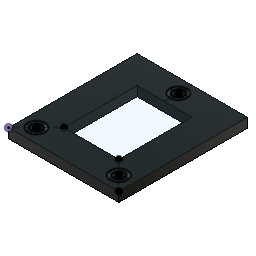
Combat Arrow Assembly v9 (Autodesk Fusion 360 archive; units mm, degrees)
design "Neoprene Clamp mk2"
Autodesk Fusion 360 part; units mm, degrees
sketch "Sketch1" plane through (0, 0, 0) normal (0, 0, 1) x (1, 0, 0)
  line L0 (0, 0) -> (38.354, 0)
  line L1 (38.354, 0) -> (38.354, 44.704)
  line L2 (38.354, 44.704) -> (0, 44.704)
  line L3 (0, 44.704) -> (0, 0)
  line L4 (28.702, 35.052) -> (9.652, 35.052)
  line L5 (9.652, 35.052) -> (9.652, 9.652)
  line L6 (9.652, 9.652) -> (28.702, 9.652)
  line L7 (28.702, 9.652) -> (28.702, 35.052)
  line L8 (28.702, 35.052) -> (9.652, 9.652) construction
  line L9 (9.652, 35.052) -> (28.702, 9.652) construction
  line L10 (19.177, 44.704) -> (19.177, 0) construction
  line L11 (0, 22.352) -> (38.354, 22.352) construction
  point P0 (19.177, 22.352)
  dimension "d13" = 38.354
  dimension "d14" = 44.704
  dimension "d15" = 19.05
  dimension "d16" = 25.4
  constraint horizontal L0
  constraint vertical L1
  constraint horizontal L2
  constraint vertical L3
  constraint coincident L0.start L3.end
  constraint horizontal L4
  constraint perpendicular L4 L5
  constraint parallel L4 L6
  constraint parallel L5 L7
  constraint coincident L8 P0
  constraint coincident L9 P0
  constraint midpoint L2 L10.start
  constraint midpoint L0 L10.end
  constraint midpoint L3 L11.start
  constraint midpoint L1 L11.end
  constraint coincident P0 L11
  constraint coincident P0 L10
  measures "d13" distance of L0.start L0.end
  measures "d14" distance of L0.start L2.end
  measures "d15" distance of L5.end L6.end
  measures "d16" distance of L4.start L6.end
extrude "Extrude1" add sketch "Sketch1" along normal blind 3.3528
sketch "Sketch2" plane through (0, 0, 3.3528) normal (0, 0, 1) x (-1, 0, 0)
  line L0 (-28.702, -35.052) -> (-28.702, -9.652)
  line L1 (-28.702, -9.652) -> (-9.652, -9.652)
  line L2 (-9.652, -9.652) -> (-9.652, -35.052)
  line L3 (-9.652, -35.052) -> (-28.702, -35.052)
  line L4 (0, -44.704) -> (0, 0)
  line L5 (0, 0) -> (-38.354, 0)
  line L6 (-38.354, 0) -> (-38.354, -44.704)
  line L7 (-38.354, -44.704) -> (0, -44.704)
  line L8 (-19.177, -35.052) -> (-19.177, -44.704) construction
  line L9 (-9.652, -9.652) -> (0, 0) construction
  line L10 (-28.702, -9.652) -> (-38.354, 0) construction
  circle A0 centre (-19.177, -39.878) radius 2.921
  circle A1 centre (-19.177, -39.878) radius 1.778
  circle A2 centre (-4.826, -4.826) radius 2.921
  circle A3 centre (-4.826, -4.826) radius 1.778
  circle A4 centre (-33.528, -4.826) radius 2.921
  circle A5 centre (-33.528, -4.826) radius 1.778
  point P0 (-19.177, -39.878)
  point P1 (-33.528, -4.826)
  point P2 (-4.826, -4.826)
  dimension "d8" = 5.842
  dimension "d9" = 3.556
  constraint midpoint L3 L8.start
  constraint midpoint L7 L8.end
  constraint coincident L1.end L2.start
  constraint coincident L4.end L5.start
  constraint coincident L0.end L1.start
  constraint coincident L5.end L6.start
  constraint midpoint L8 P0
  constraint midpoint L10 P1
  constraint midpoint L9 P2
  constraint coincident P0 A0.centre
  constraint coincident P2 A2.centre
  constraint coincident P1 A4.centre
  constraint concentric A4 A5
  constraint equal A0 A2
  constraint equal A1 A3
  constraint equal A3 A5
  constraint equal A2 A4
  measures "d8" diameter of A0
  measures "d9" diameter of A1
extrude "Extrude2" cut sketch "Sketch2" against normal through all contours A1 | A3 | A5
extrude "Extrude3" cut sketch "Sketch2" against normal blind 2.286 contours A0 | A2 | A4
